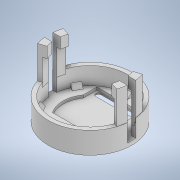
# Autodesk Inventor part: motor-case-encoder
Saved by Autodesk Inventor 2020.1 (Build 241239000, 239)
## iProperties
Created: 2019-10-08
Part Number: motor-case-encoder
Material: Genérico
Document SubType Name: Modeling
Designer: rotje
Density: 1 g/cm^3
Appearance: Valor por defecto
Author: rotje
Autodesk Inventor part; units mm, degrees
ref_plane "YZ Plane" through (0, 0, 0) normal (1, 0, 0) x (0, 1, 0)
ref_plane "XZ Plane" through (0, 0, 0) normal (0, 1, 0) x (-1, 0, 0)
ref_plane "XY Plane" through (0, 0, 0) normal (0, 0, 1) x (1, 0, 0)
sketch "Boceto1" plane through (0, 0, 0) normal (0, 1, 0) x (-1, 0, 0)
  circle A0 centre (0, 0) radius 15.5
  dimension "d0" = 31
  constraints: 1 centre point, 1 coincident
  measures "d0" diameter of A0
extrude "Extrusión1" add sketch "Boceto1" along normal blind 1.5
sketch "Boceto2" plane through (0, 1.5, 0) normal (0, 1, 0) x (1, 0, 0)
  line L0 (8.2045, 10.7962) -> (-8.2045, 10.7962)
  line L1 (-8.2045, -5.7138) -> (8.2045, -5.7138)
  line L2 (-8.2045, 10.7962) -> (-8.2045, 5.7172)
  line L3 (8.2045, 10.7962) -> (8.2045, 5.7172)
  line L4 (8.2045, 10.7962) -> (8.2045, 5.7172)
  line L5 (-8.2045, -5.7138) -> (-8.2068, -5.7138)
  line L6 (8.2045, -5.7138) -> (8.2068, -5.7138)
  arc A0 (-8.2045, 5.7172) -> (-8.2068, -5.7138) centre (0, 0) ccw
  arc A1 (8.2068, -5.7138) -> (8.2045, 5.7172) centre (0, 0) ccw
  line L7 (8.2045, 5.7172) -> (8.2045, 10.7962)
  line L8 (-8.2045, 10.7962) -> (-8.2045, 5.7172)
  constraints: 18 end point, 4 point on circle, 3 horizontal, 2 centre point, 2 parallel, 1 coincident, 1 perpendicular
extrude "Extrusión2" cut sketch "Boceto2" against normal blind 1.016
sketch "Boceto3" plane through (0, 1.5, 0) normal (0, 1, 0) x (1, 0, 0)
  circle A0 centre (0, 0) radius 15.5 projected
  line L0 (-0.0853, 15.4998) -> (-0.0853, -15.4998)
  line L1 (0, 0) -> (-0.0853, -1.4976)
  line L2 (13.9232, -1.4646) -> (15.4223, -1.55)
  line L3 (0, 0) -> (-0.0853, 1.4976)
  line L4 (13.9194, 1.5) -> (15.4187, 1.5854)
  line L5 (-13.914, 1.5494) -> (-15.4223, 1.55)
  arc A1 (-13.9139, -1.55) -> (13.9232, -1.4646) centre (0, 0) ccw
  arc A2 (13.9194, 1.5) -> (-13.914, 1.5494) centre (0, 0) ccw
  arc A3 (-15.4223, -1.55) -> (15.4223, -1.55) centre (0, 0) ccw
  arc A4 (15.4187, 1.5854) -> (-15.4223, 1.55) centre (0, 0) ccw
  line L6 (-15.4223, -1.55) -> (-13.9139, -1.55)
  dimension "d15" = 1.5
  dimension "d16" = 1.5
  dimension "d31" = 14
  dimension "d32" = 14
  constraints: 15 point on circle, 14 end point, 4 centre point, 2 coincident, 2 perpendicular, 2 point on line, 1 horizontal, 1 vertical
  measures "d15" distance of L1.start L1.end
  measures "d16" distance of L1.start L3.end
  measures "d31" radius of A2
  measures "d32" radius of A1
extrude "Extrusión3" add sketch "Boceto3" along normal blind 6.516 contours L4 A2 L0 A0 | A0 L0 A1 L2 | L0 A2 L5 A0 | A0 L6 A1 L0
sketch "Boceto4" plane through (0, 0.484, 0) normal (0, 1, 0) x (1, 0, 0)
  line L0 (8.2045, 10.7962) -> (8.2045, 5.7172) projected
  line L1 (8.2045, 10.7962) -> (6.3495, 10.7962)
  line L2 (-8.2045, 10.7962) -> (8.2045, 10.7962) projected
  line L3 (6.3495, 10.7962) -> (6.3495, 9.5262)
  circle A0 centre (6.3495, 9.5262) radius 1
  circle A1 centre (3.8095, 9.5262) radius 1
  circle A2 centre (1.2695, 9.5262) radius 1
  circle A3 centre (-1.2705, 9.5262) radius 1
  circle A4 centre (-3.8105, 9.5262) radius 1
  circle A5 centre (-6.3505, 9.5262) radius 1
  line L4 (-6.3505, 10.5262) -> (6.3495, 10.5262)
  line L5 (-6.3505, 8.5262) -> (6.3495, 8.5262)
  point P0 (0, 0)
  point P1 (3.8095, 8.5262)
  point P2 (3.8095, 10.5262)
  point P3 (1.2695, 8.5262)
  point P4 (1.2695, 10.5262)
  point P5 (-1.2705, 8.5262)
  point P6 (-1.2705, 10.5262)
  point P7 (-3.8105, 8.5262)
  point P8 (-3.8105, 10.5262)
  dimension "d19" = 1.855
  dimension "d20" = 1.27
  dimension "d21" = 2
  dimension "d27" = 2.54
  constraints: 8 end point, 6 centre point, 4 point on circle, 2 horizontal, 2 point on line, 1 coincident, 1 perpendicular, 10 other
  measures "d19" distance of L0.start L1.end
  measures "d20" distance of L1.end L3.end
  measures "d21" diameter of A0
  measures "d27" distance of A0.centre A1.centre
extrude "Extrusión4" cut sketch "Boceto4" against normal blind 0.984
sketch "Boceto7" plane through (0, 1.5, 0) normal (0, 1, 0) x (1, 0, 0)
  arc A0 (-13.9139, -1.55) -> (13.9232, -1.4646) centre (0, 0) ccw projected
  line L0 (0, -12.5) -> (1.5, -12.5)
  line L1 (1.5, -12.5) -> (-1.5, -12.5)
  line L2 (-1.5, -12.5) -> (-1.5, -14)
  line L3 (1.5, -12.5) -> (1.5, -14)
  line L4 (-11.5753, -4.951) -> (-12.8744, -5.701)
  line L5 (-10.0753, -7.549) -> (-11.5753, -4.951)
  line L6 (-10.0753, -7.549) -> (-11.3744, -8.299)
  line L7 (-10.0753, 7.549) -> (-11.3744, 8.299)
  line L8 (-11.5753, 4.951) -> (-10.0753, 7.549)
  line L9 (-11.5753, 4.951) -> (-12.8744, 5.701)
  line L10 (1.5, 12.5) -> (1.5, 14)
  line L11 (-1.5, 12.5) -> (1.5, 12.5)
  line L12 (-1.5, 12.5) -> (-1.5, 14)
  line L13 (11.5753, 4.951) -> (12.8744, 5.701)
  line L14 (10.0753, 7.549) -> (11.5753, 4.951)
  line L15 (10.0753, 7.549) -> (11.3744, 8.299)
  line L16 (10.0753, -7.549) -> (11.3744, -8.299)
  line L17 (11.5753, -4.951) -> (10.0753, -7.549)
  line L18 (11.5753, -4.951) -> (12.8744, -5.701)
  circle A1 centre (0, 0) radius 14
  point P0 (1.5, 13.9194)
  point P1 (-1.5, 13.9194)
  point P2 (12.8046, 5.6607)
  point P3 (11.3046, 8.2587)
  point P4 (11.3046, -8.2587)
  point P5 (12.8046, -5.6607)
  point P6 (1.5, -13.9194)
  point P7 (-1.5, -13.9194)
  point P8 (-12.8046, -5.6607)
  point P9 (-11.3046, -8.2587)
  point P10 (-11.3046, 8.2587)
  point P11 (-12.8046, 5.6607)
  dimension "d55" = 360
  dimension "d57" = 28
  constraints: 38 end point, 1 centre point, 1 coincident, 1 perpendicular, 1 point on line, 1 vertical, 49 other
  measures "d57" diameter of A1
extrude "Extrusión6" add sketch "Boceto7" along normal blind 1.5 contours L4 L5 L6 A0 | A1 L7 L8 L9 | L2 L1 L0 L3 A0 | A1 L10 L11 L12 | L16 L17 L18 A0 | A1 L13 L14 L15
chamfer "Chaflán3" distance 1.49 angle 45 6 edges at (-10.8253, 3, -6.25) (0, 3, -12.5) (10.8253, 3, -6.25) (-10.8253, 3, 6.25) (10.8253, 3, 6.25) (0, 3, 12.5)
sketch "Boceto12" plane through (0, 0, 0) normal (0, 0, 1) x (1, 0, 0)
  line L0 (-15.4223, 1.5) -> (-15.4223, 8.016) projected
  line L1 (-15.4223, 8.016) -> (-15.4223, 20.056)
  line L2 (-15.4223, 20.056) -> (-11.9223, 20.056)
  line L3 (-11.9223, 20.056) -> (-11.9223, 16.056)
  line L4 (-11.9223, 16.056) -> (-13.9803, 16.056)
  line L5 (-13.9803, 16.056) -> (-13.9803, 8.016)
  line L6 (-15.4223, 9.7192) -> (-15.4223, 6.3361)
  line L7 (-15.4223, 6.3361) -> (-13.9803, 6.3361)
  line L8 (-13.9803, 6.3361) -> (-13.9803, 8.016)
  line L9 (0, 0) -> (0, 19.2714)
  line L10 (15.4223, 1.5) -> (15.4223, 8.016)
  line L11 (15.4223, 8.016) -> (15.4223, 20.056)
  line L12 (15.4223, 20.056) -> (11.9223, 20.056)
  line L13 (11.9223, 20.056) -> (11.9223, 16.056)
  line L14 (11.9223, 16.056) -> (13.9803, 16.056)
  line L15 (13.9803, 16.056) -> (13.9803, 8.016)
  line L16 (15.4223, 9.7192) -> (15.4223, 6.3361)
  line L17 (15.4223, 6.3361) -> (13.9803, 6.3361)
  line L18 (13.9803, 6.3361) -> (13.9803, 8.016)
  dimension "d67" = 12.04
  dimension "d68" = 3.5
  dimension "d69" = 4
  dimension "d70" = 2.058
  constraints: 36 end point, 10 symmetric about line, 5 perpendicular, 4 point on line, 2 vertical, 1 horizontal
  measures "d67" distance of L0.end L1.end
  measures "d68" distance of L1.end L2.end
  measures "d69" distance of L2.end L3.end
  measures "d70" distance of L3.end L4.end
revolve "Revolución1" add sketch "Boceto12" angle 18 about axis through (0, 0, 0) along (0, 1, 0) and the other way 18
sketch "Boceto13" plane through (0, 1.5, 0) normal (0, 1, 0) x (1, 0, 0)
  circle A0 centre (0, 0) radius 15.5
  arc A1 (13.9194, 1.5) -> (-13.3148, 4.3262) centre (0, 0) ccw projected
  circle A2 centre (0, 0) radius 14
  line L0 (-15.4223, -1.55) -> (-13.9139, -1.55) projected
  line L1 (-13.9139, -1.55) -> (-15.4223, -1.55)
  line L2 (-13.9139, 1.55) -> (-15.4223, 1.55)
  constraints: 4 end point, 2 centre point, 2 coincident, 2 point on circle, 1 collinear, 1 horizontal
extrude "Extrusión8" cut sketch "Boceto13" along normal blind 20 contours L2 A2 L0 A0
sketch "Boceto14" plane through (0, 20.056, 0) normal (0, 1, 0) x (1, 0, 0)
  line L0 (-15.4223, -1.55) -> (-13.9139, -1.55) projected
  line L1 (-13.9139, -1.55) -> (-11.8211, -1.55)
  arc A0 (-11.3388, 3.6842) -> (-11.3388, -3.6842) centre (0, 0) ccw projected
  arc A1 (-13.9139, 1.55) -> (-13.9139, -1.55) centre (0, 0) ccw projected
  line L2 (-13.9139, 1.55) -> (-11.8211, 1.55)
  line L3 (-13.9139, 1.55) -> (-15.4223, 1.55) projected
  line L4 (-11.8211, 1.55) -> (-15.4223, 1.55)
  line L5 (-13.9139, -1.55) -> (-15.4223, -1.55)
  circle A2 centre (0, 0) radius 15.5
  circle A3 centre (0, 0) radius 11.9223
  line L6 (0, -3.1566) -> (0, 2.4936)
  line L7 (15.4223, -1.55) -> (13.9139, -1.55)
  line L8 (13.9139, -1.55) -> (11.8211, -1.55)
  arc A4 (13.9139, -1.55) -> (13.9139, 1.55) centre (0, 0) ccw
  line L9 (13.9139, 1.55) -> (11.8211, 1.55)
  line L10 (13.9139, 1.55) -> (15.4223, 1.55)
  line L11 (11.8211, 1.55) -> (15.4223, 1.55)
  line L12 (13.9139, -1.55) -> (15.4223, -1.55)
  point P0 (-15.4223, 1.55)
  point P1 (-15.4223, -1.55)
  constraints: 22 end point, 6 symmetric about line, 3 centre point, 3 horizontal, 3 point on circle, 2 coincident, 1 collinear, 1 vertical, 1 other
extrude "Extrusión9" cut sketch "Boceto14" against normal blind 15 contours A2 L3 A1 L0 | A1 L2 A0 L1 | L7 A4 L10 A2 | L8 A3 L9 A4
sketch "Boceto15" plane through (0, 0, 0) normal (0, 0, 1) x (1, 0, 0)
  line L0 (-13.2961, 16.056) -> (-11.3388, 16.056) projected
  line L1 (-12.6577, 16.056) -> (-9.3722, 16.056)
  line L2 (-9.3722, 16.056) -> (-9.3722, 20.522)
  line L3 (-9.3722, 20.522) -> (-12.6577, 20.522)
  line L4 (-12.6577, 20.522) -> (-12.6577, 16.056)
  line L5 (0, 24.1965) -> (0, 13.5)
  point P0 (0, 0)
  constraints: 10 end point, 3 perpendicular, 1 collinear, 1 point on line, 1 vertical
revolve "Revolución2" cut sketch "Boceto15" angle 360 about axis through (0, 24.1965, 0) along (0, -1, 0)
